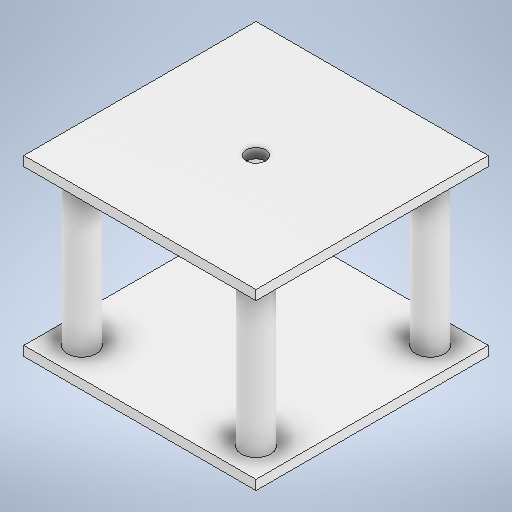
# Autodesk Inventor part: Central_base
Saved by Autodesk Inventor 2025.3 (Build 293356000, 356)
## iProperties
Created: 2025-07-26
Part Number: Central_base
Material: Plástico ABS
Document SubType Name: Modeling
Designer: KEVIN
Density: 1.06 g/cm^3
Appearance: Suave - Blanco
Mass: 298.442 g
Surface Area: 1096.66 cm^2
Volume: 281.549 cm^3
Author: KEVIN
Autodesk Inventor part; units mm, degrees
ref_plane "YZ Plane" through (0, 0, 0) normal (1, 0, 0) x (0, 1, 0)
ref_plane "XZ Plane" through (0, 0, 0) normal (0, 1, 0) x (-1, 0, 0)
ref_plane "XY Plane" through (0, 0, 0) normal (0, 0, 1) x (1, 0, 0)
sketch "Boceto1" plane through (0, 0, 0) normal (0, 1, 0) x (-1, 0, 0)
  line L0 (60, -60) -> (-60, -60)
  line L1 (-60, -60) -> (-60, 60)
  line L2 (-60, 60) -> (60, 60)
  line L3 (60, 60) -> (60, -60)
  line L4 (60, -60) -> (-60, 60) construction
  line L5 (-60, -60) -> (60, 60) construction
  point P0 (0, 0)
  dimension "d0" = 120
  dimension "d1" = 120
  constraints: 12 end point, 2 midpoint, 2 parallel, 1 horizontal, 1 perpendicular
  measures "d0" distance of L1.end L2.end
  measures "d1" distance of L0.end L1.end
extrude "Extrusión1" add sketch "Boceto1" along normal blind 5
sketch "Boceto2" plane through (0, 5, 0) normal (0, 1, 0) x (1, 0, 0)
  line L0 (45, -45) -> (-45, -45)
  line L1 (-45, -45) -> (-45, 45)
  line L2 (-45, 45) -> (45, 45)
  line L3 (45, 45) -> (45, -45)
  line L4 (45, -45) -> (-45, 45) construction
  line L5 (-45, -45) -> (45, 45) construction
  circle A0 centre (-45, 45) radius 7.5
  circle A1 centre (45, 45) radius 7.5
  circle A2 centre (-45, -45) radius 7.5
  circle A3 centre (45, -45) radius 7.5
  point P0 (0, 0)
  dimension "d4" = 90
  dimension "d5" = 90
  dimension "d6" = 15
  dimension "d7" = 15
  dimension "d8" = 15
  dimension "d9" = 15
  constraints: 12 end point, 4 centre point, 4 coincident, 2 midpoint, 2 parallel, 1 horizontal, 1 perpendicular
  measures "d4" distance of L1.end L2.end
  measures "d5" distance of L0.end L1.end
  measures "d6" diameter of A0
  measures "d7" diameter of A1
  measures "d8" diameter of A2
  measures "d9" diameter of A3
extrude "Extrusión2" add sketch "Boceto2" along normal blind 80 contours A2 L1 L0 | L0 L1 A2 | A3 L3 L0 | L0 L3 A3 | A0 L2 L1 | L1 L2 A0 | A1 L2 L3 | L3 L2 A1
sketch "Boceto3" plane through (-45, 85, 45) normal (0, 1, 0) x (1, 0, 0)
  circle A0 centre (90, 90) radius 7.5 projected
  line L0 (90, 90) -> (-30, 90)
  line L1 (-30, 90) -> (-30, -30)
  line L2 (-30, -30) -> (90, -30)
  line L3 (90, -30) -> (90, 90)
  line L4 (-15, 105) -> (105, 105)
  line L5 (105, 105) -> (105, -15)
  line L6 (105, -15) -> (-15, -15)
  line L7 (-15, -15) -> (-15, 105)
  line L8 (-15, 105) -> (105, -15) construction
  line L9 (105, 105) -> (-15, -15) construction
  point P0 (45, 45)
  dimension "d12" = 120
  dimension "d13" = 120
  constraints: 20 end point, 4 parallel, 2 horizontal, 2 midpoint, 2 perpendicular
  measures "d12" distance of L5.end L6.end
  measures "d13" distance of L4.end L5.end
extrude "Extrusión3" add sketch "Boceto3" along normal blind 5 contours A0 L3 L0 | A0 L0 L7 L4 L5 L6 L3 | L0 L3 A0 | A0 L3 L6 L7 L0
sketch "Boceto4" plane through (-45, 90, 45) normal (0, 1, 0) x (1, 0, 0)
  circle A0 centre (45, 45) radius 5
  dimension "d16" = 10
  constraints: 1 centre point, 1 coincident
  measures "d16" diameter of A0
extrude "Extrusión4" cut sketch "Boceto4" against normal blind 10
